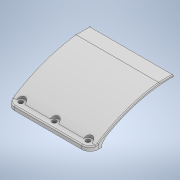
# Autodesk Inventor part: Wheel Shield
Saved by Autodesk Inventor 2020 (Build 240168000, 168)
## iProperties
Created: 2020-02-22
Part Number: Wheel Shield
Material: Generic
Document SubType Name: Modeling
Designer: maple
Density: 1 g/cm^3
Appearance: Default
Author: maple
Autodesk Inventor part; units mm, degrees
ref_plane "YZ Plane" through (0, 0, 0) normal (1, 0, 0) x (0, 1, 0)
ref_plane "XZ Plane" through (0, 0, 0) normal (0, 1, 0) x (-1, 0, 0)
ref_plane "XY Plane" through (0, 0, 0) normal (0, 0, 1) x (1, 0, 0)
sketch "Sketch1" plane through (0, 0, 0) normal (0, 1, 0) x (-1, 0, 0)
  line L0 (0, 0) -> (-101.6, 0)
  line L1 (-101.6, 0) -> (-101.6, -101.6)
  line L2 (-101.6, -101.6) -> (0, -101.6)
  line L3 (0, -101.6) -> (0, 0)
  dimension "d0" = 101.6
  dimension "d1" = 101.6
  constraints: 8 end point, 2 parallel, 1 horizontal, 1 perpendicular
  measures "d0" distance of L2.end L1.end
  measures "d1" distance of L1.end L0.end
extrude "Extrusion1" add sketch "Sketch1" along normal blind 33.02
sketch "Sketch2" plane through (101.6, 0, 0) normal (1, 0, 0) x (0, 0, -1)
  line L0 (0, 0) -> (101.6, 0) projected
  line L1 (0, 0) -> (0, 5.08)
  line L2 (0, 0) -> (0, 33.02) projected
  line L3 (0, 5.08) -> (7.62, 5.08)
  line L4 (0, 33.02) -> (101.6, 33.02) projected
  line L5 (101.6, 33.02) -> (101.6, 29.972)
  line L6 (101.6, 0) -> (101.6, 33.02) projected
  line L7 (7.62, 5.08) -> (11.43, 5.08)
  line L8 (101.6, 33.02) -> (83.82, 33.02)
  arc A0 (83.82, 33.02) -> (7.62, 5.08) centre (105.8024, -144.8111) ccw
  line L9 (11.43, 5.08) -> (15.24, 5.08)
  line L10 (15.24, 5.08) -> (15.24, 0)
  arc A1 (101.6, 29.972) -> (15.24, 5.08) centre (99.7421, -125.8363) ccw
  arc A2 (22.163, 9.2976) -> (15.24, 2.54) centre (35.2283, -11.0126) ccw
  dimension "d4" = 5.08
  dimension "d5" = 7.62
  dimension "d6" = 3.048
  dimension "d7" = 3.81
  dimension "d8" = 17.78
  dimension "d9" = 3.81
  constraints: 14 end point, 7 point on circle, 4 point on line, 3 centre point, 2 horizontal, 2 perpendicular, 1 midpoint
  measures "d4" distance of L0.start L1.end
  measures "d5" distance of L1.end L3.end
  measures "d6" distance of L4.end L5.end
  measures "d7" distance of L3.end L7.end
  measures "d8" distance of L4.end L8.end
  measures "d9" distance of L7.end L9.end
extrude "Extrusion2" cut sketch "Sketch2" against normal blind 101.6 contours L10 A2 A1 L6 L0 | L2 L4 A0 L3
sketch "Sketch3" plane through (101.6, 5.08, 0) normal (0, 1, 0) x (1, 0, 0)
  line L0 (0, 7.62) -> (-101.6, 7.62) projected
  line L1 (-101.6, 7.62) -> (-91.44, 7.62)
  line L2 (0, 7.62) -> (0, 83.82) projected
  line L3 (0, 7.62) -> (-10.16, 7.62)
  circle A0 centre (-91.44, 7.62) radius 5.08
  circle A1 centre (-50.8, 7.62) radius 5.08
  circle A2 centre (-10.16, 7.62) radius 5.08
  point P0 (-101.6, 0)
  dimension "d12" = 10.16
  dimension "d13" = 10.16
  dimension "d14" = 10.16
  dimension "d15" = 10.16
  dimension "d16" = 10.16
  constraints: 4 end point, 3 centre point, 2 coincident, 2 point on line, 1 midpoint
  measures "d12" distance of L0.end L1.end
  measures "d13" distance of L0.start L3.end
  measures "d14" diameter of A0
  measures "d15" diameter of A1
  measures "d16" diameter of A2
extrude "Extrusion3" cut sketch "Sketch3" along normal blind 101.6
sketch "Sketch4" plane through (101.6, 5.08, 0) normal (0, 1, 0) x (1, 0, 0)
  line L0 (-96.52, 7.62) -> (-101.6, 7.62) projected
  line L1 (-101.6, 7.62) -> (-91.44, 7.62)
  line L2 (0, 7.62) -> (0, 0) projected
  line L3 (0, 7.62) -> (-10.16, 7.62)
  circle A0 centre (-91.44, 7.62) radius 2.54
  line L4 (-55.88, 7.62) -> (-86.36, 7.62) projected
  line L5 (-55.88, 7.62) -> (-50.8, 7.62)
  circle A1 centre (-50.8, 7.62) radius 2.54
  circle A2 centre (-10.16, 7.62) radius 2.54
  point P0 (-101.6, 0)
  dimension "d19" = 10.16
  dimension "d20" = 10.16
  dimension "d21" = 5.08
  dimension "d22" = 5.08
  dimension "d23" = 5.08
  dimension "d24" = 5.08
  constraints: 6 end point, 3 centre point, 3 coincident, 3 horizontal
  measures "d19" distance of L0.end L1.end
  measures "d20" distance of L2.start L3.end
  measures "d21" diameter of A0
  measures "d22" distance of L4.start L5.end
  measures "d23" diameter of A1
  measures "d24" diameter of A2
extrude "Extrusion4" cut sketch "Sketch4" against normal blind 101.6
fillet "Fillet1" radius 10.16 2 edges at (0, 2.54, 0) (101.6, 2.54, 0)
fillet "Fillet2" radius 1.27 7 edges at (3.9383, 5.08, -2.1278) (97.6617, 5.08, -2.1278) (50.8, 5.08, 0) (50.8, 33.02, -101.6) (50.8, 29.972, -101.6) (0, 1.27, -15.24) (101.6, 1.27, -15.24)
fillet "Fillet3" radius 1.016 12 edges at (101.5182, 5.8937, -8.8737) (100.9717, 4.4352, -6.6426) (101.6, 23.9349, -45.5371) (101.6, 24.7978, -59.8791) (101.6, 1.5089, -14.5784) (101.6, 6.269, -18.3596) (0, 24.7978, -59.8791) (0.0818, 5.8937, -8.8737) (0.6283, 4.4352, -6.6426) (0, 23.9349, -45.5371) (0, 6.269, -18.3596) (0, 1.5089, -14.5784)
body "Solid1"
